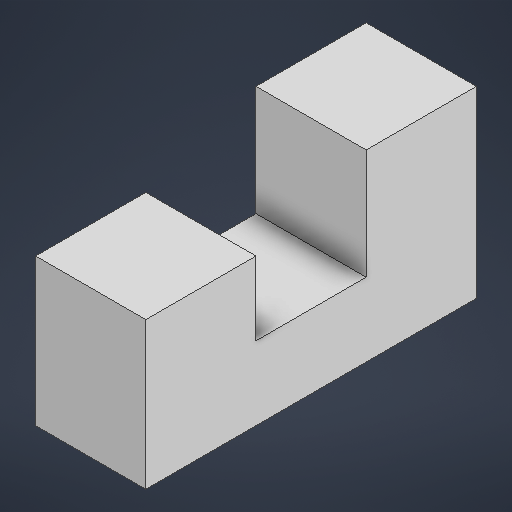
# Autodesk Inventor part: Part2
Saved by Autodesk Inventor 2026 (Build 300175050, 175E)
## iProperties
Created: 2026-03-12
Part Number: Part2
Material: Generic
Document SubType Name: Modeling
Designer: Administrator
Density: 1 g/cm^3
Appearance: Default
Author: Administrator
Autodesk Inventor part; units mm, degrees
ref_plane "YZ Plane" through (0, 0, 0) normal (1, 0, 0) x (0, 1, 0)
ref_plane "XZ Plane" through (0, 0, 0) normal (0, 1, 0) x (-1, 0, 0)
ref_plane "XY Plane" through (0, 0, 0) normal (0, 0, 1) x (1, 0, 0)
sketch "Sketch1" plane through (0, 0, 0) normal (1, 0, 0) x (0, 1, 0)
  line L0 (0, 0) -> (25, 0)
  line L1 (25, 0) -> (25, -45)
  line L2 (25, -45) -> (0, -45)
  line L3 (0, -45) -> (0, 0)
  dimension "d0" = 45
  dimension "d1" = 25
  constraints: 8 end point, 2 parallel, 1 horizontal, 1 perpendicular
  measures "d0" distance of L0.end L1.end
  measures "d1" distance of L1.end L2.end
extrude "Extrusion1" add sketch "Sketch1" along normal mid plane 15
sketch "Sketch7" plane through (7.5, 0, 0) normal (1, 0, 0) x (0, 0, -1)
  line L0 (15, 31.5845) -> (30, 31.5845)
  line L1 (30, 31.5845) -> (30, 10)
  line L2 (30, 10) -> (15, 10)
  line L3 (15, 10) -> (15, 31.5845)
  line L4 (45, 0) -> (45, 25) projected
  line L5 (0, 25) -> (0, 0) projected
  line L6 (0, 0) -> (45, 0) projected
  dimension "d10" = 15
  dimension "d12" = 15
  dimension "d15" = 15
  dimension "d16" = 10
  constraints: 8 end point, 2 parallel, 1 horizontal, 1 perpendicular
  measures "d10" distance between parallel lines of L4 L1
  measures "d12" distance of L0.start L0.end
  measures "d15" distance between parallel lines of L5 L3
  measures "d16" distance between parallel lines of L6 L2
extrude "Extrusion2" cut sketch "Sketch7" against normal through all
sketch "Sketch9" plane through (7.5, 0, 0) normal (1, 0, 0) x (0, 0, -1)
  line L0 (-4.7353, 35) -> (15.2647, 35)
  line L1 (15.2647, 35) -> (15.2647, 20)
  line L2 (15.2647, 20) -> (-4.7353, 20)
  line L3 (-4.7353, 20) -> (-4.7353, 35)
  line L4 (0, 0) -> (45, 0) projected
  dimension "d20" = 15
  dimension "d21" = 20
  dimension "d22" = 20
  constraints: 8 end point, 2 parallel, 1 horizontal, 1 perpendicular
  measures "d20" distance between parallel lines of L2 L0
  measures "d21" distance of L0.start L0.end
  measures "d22" distance between parallel lines of L4 L2
extrude "Extrusion3" cut sketch "Sketch9" against normal through all
body "Solid1"
